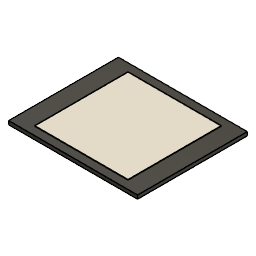
InkTime_Asamblare_Fin (Autodesk Fusion 360 archive; units mm, degrees)
design "EPD_DISPLAY"
part number: 2026-03-23-13-23-22-558
Autodesk Fusion 360 part; units mm, degrees
box "BoxPrimitive2" add length 31.8 width 37.32 height 1.05 placed x (0, 0, 1) y (1, 0, 0) z (0, 1, 0) at (-13, 0, 3) makes body 1
move_body "Move1" bodies 1 to x (1, 0, 0) y (0, 1, 0) z (0, 0, 1) at (-5.66, 0, -18.9)
box "BoxPrimitive3" add length 27 width 27 height 0.1 placed x (0, 0, 1) y (1, 0, 0) z (0, 1, 0) at (26, 1.05, 40) separate body makes body 2
move_body "Move2" bodies 2 to x (1, 0, 0) y (0, 1, 0) z (0, 0, 1) at (-39.5, -0.1, -53.5)
move_body "Move3" bodies 2 to x (1, 0, 0) y (0, 1, 0) z (0, 0, 1) at (0, 0.1, 0)
